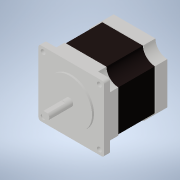
# Autodesk Inventor part: MC18_Motor
Saved by Autodesk Inventor 2021 (Build 250183000, 183)
## iProperties
Created: 2020-01-08
Part Number: MC18_Motor
Material: Generisch
Document SubType Name: Modeling
Designer: kaebi
Density: 1 g/cm^3
Appearance: Vorgabe
Description: Schrittmotor M-2222-3.0S
Stock Number: -
Author: kaebi
Autodesk Inventor part; units mm, degrees
ref_plane "YZ Plane" through (0, 0, 0) normal (1, 0, 0) x (0, 1, 0)
ref_plane "XZ Plane" through (0, 0, 0) normal (0, 1, 0) x (-1, 0, 0)
ref_plane "XY Plane" through (0, 0, 0) normal (0, 0, 1) x (1, 0, 0)
sketch "Skizze1" plane through (0, 0, 0) normal (0, 0, 1) x (1, 0, 0)
  line L0 (-27.5, -27.5) -> (27.5, -27.5)
  line L1 (27.5, -27.5) -> (27.5, 27.5)
  line L2 (27.5, 27.5) -> (-27.5, 27.5)
  line L3 (-27.5, 27.5) -> (-27.5, -27.5)
  line L4 (-27.5, -27.5) -> (27.5, 27.5) construction
  line L5 (27.5, -27.5) -> (-27.5, 27.5) construction
  point P0 (0, 0)
  dimension "d0" = 55
  dimension "d1" = 55
  constraints: 12 end point, 2 midpoint, 2 parallel, 1 horizontal, 1 perpendicular
  measures "d0" distance of L2.end L1.end
  measures "d1" distance of L1.end L0.end
extrude "Extrusion1" add sketch "Skizze1" against normal blind 12
sketch "Skizze2" plane through (0, 0, -12) normal (0, 0, -1) x (-1, 0, 0)
  line L0 (27.5, 27.5) -> (-27.5, 27.5) projected
  circle A0 centre (-27.5, 27.5) radius 10
  line L1 (27.5, -27.5) -> (27.5, 27.5) projected
  circle A1 centre (27.5, 27.5) radius 10
  circle A2 centre (27.5, -27.5) radius 10
  circle A3 centre (-27.5, -27.5) radius 10
  point P0 (0, 0)
  dimension "d4" = 20
  constraints: 4 centre point, 3 coincident, 3 equal radius
  measures "d4" diameter of A0
extrude "Extrusion2" cut sketch "Skizze2" against normal blind 7
sketch "Skizze3" plane through (0, 0, -12) normal (0, 0, -1) x (-1, 0, 0)
  arc A0 (27.5, -17.5) -> (17.5, -27.5) centre (27.5, -27.5) ccw projected
  line L0 (27.5, -17.5) -> (27.5, 17.5) projected
  arc A1 (17.5, 27.5) -> (27.5, 17.5) centre (27.5, 27.5) ccw projected
  line L1 (17.5, 27.5) -> (-17.5, 27.5) projected
  arc A2 (-27.5, 17.5) -> (-17.5, 27.5) centre (-27.5, 27.5) ccw projected
  line L2 (-27.5, 17.5) -> (-27.5, -17.5) projected
  arc A3 (-17.5, -27.5) -> (-27.5, -17.5) centre (-27.5, -27.5) ccw projected
  line L3 (-17.5, -27.5) -> (17.5, -27.5) projected
  line L4 (-17.0119, 27) -> (17.0119, 27)
  arc A4 (17.0119, 27) -> (27, 17.0119) centre (27.5, 27.5) ccw
  line L5 (27, 17.0119) -> (27, -17.0119)
  arc A5 (27, -17.0119) -> (17.0119, -27) centre (27.5, -27.5) ccw
  line L6 (17.0119, -27) -> (-17.0119, -27)
  arc A6 (-17.0119, -27) -> (-27, -17.0119) centre (-27.5, -27.5) ccw
  line L7 (-27, -17.0119) -> (-27, 17.0119)
  arc A7 (-27, 17.0119) -> (-17.0119, 27) centre (-27.5, 27.5) ccw
  point P0 (0, 0)
  dimension "d7" = 0.5
  constraints: 8 end point, 8 point on circle, 4 centre point, 7 other
  measures "d7" distance between parallel lines of L1 L4
extrude "Extrusion3" add sketch "Skizze3" along normal blind 31 contours L4 A4 L5 A5 L6 A6 L7 A7
sketch "Skizze4" plane through (0, 0, -43) normal (0, 0, -1) x (-1, 0, 0)
  arc A0 (17.0119, 27) -> (27, 17.0119) centre (27.5, 27.5) ccw projected
  line L0 (27, 17.0119) -> (27, -17.0119) projected
  arc A1 (27, -17.0119) -> (17.0119, -27) centre (27.5, -27.5) ccw projected
  line L1 (17.0119, -27) -> (-17.0119, -27) projected
  arc A2 (-17.0119, -27) -> (-27, -17.0119) centre (-27.5, -27.5) ccw projected
  line L2 (-27, -17.0119) -> (-27, 17.0119) projected
  arc A3 (-27, 17.0119) -> (-17.0119, 27) centre (-27.5, 27.5) ccw projected
  line L3 (-17.0119, 27) -> (17.0119, 27) projected
  arc A4 (27.5, -17.5) -> (17.5, -27.5) centre (27.5, -27.5) ccw projected
  line L4 (27.5, -17.5) -> (27.5, 17.5) projected
  arc A5 (17.5, 27.5) -> (27.5, 17.5) centre (27.5, 27.5) ccw projected
  line L5 (17.5, 27.5) -> (-17.5, 27.5) projected
  arc A6 (-27.5, 17.5) -> (-17.5, 27.5) centre (-27.5, 27.5) ccw projected
  line L6 (-27.5, 17.5) -> (-27.5, -17.5) projected
  arc A7 (-17.5, -27.5) -> (-27.5, -17.5) centre (-27.5, -27.5) ccw projected
  line L7 (-17.5, -27.5) -> (17.5, -27.5) projected
  point P0 (0, 0)
extrude "Extrusion4" add sketch "Skizze4" along normal blind 10 contours A0 L0 A1 L1 A2 L2 A3 L3 | A4 L7 A7 L6 A6 L5 A5 L4
sketch "Skizze6" plane through (0, 0, 0) normal (0, 0, 1) x (1, 0, 0)
  line L0 (-23.55, -23.55) -> (23.55, -23.55)
  line L1 (23.55, -23.55) -> (23.55, 23.55)
  line L2 (23.55, 23.55) -> (-23.55, 23.55)
  line L3 (-23.55, 23.55) -> (-23.55, -23.55)
  line L4 (-23.55, -23.55) -> (23.55, 23.55) construction
  line L5 (23.55, -23.55) -> (-23.55, 23.55) construction
  circle A0 centre (-23.55, 23.55) radius 2
  circle A1 centre (23.55, 23.55) radius 2
  circle A2 centre (23.55, -23.55) radius 2
  circle A3 centre (-23.55, -23.55) radius 2
  point P0 (0, 0)
  dimension "d12" = 4
  dimension "d13" = 47.1
  dimension "d14" = 47.1
  constraints: 12 end point, 4 centre point, 4 coincident, 3 equal radius, 2 midpoint, 2 parallel, 1 horizontal, 1 perpendicular
  measures "d12" diameter of A0
  measures "d13" distance of L1.end L2.end
  measures "d14" distance of L0.end L1.end
extrude "Extrusion5" cut sketch "Skizze6" along normal through all both and the other way through all contours L3 A3 L0 | L0 A3 L3 | A2 L1 L0 | L0 L1 A2 | A0 L2 L3 | L3 L2 A0 | A1 L2 L1 | L1 L2 A1
fillet "Rundung1" radius 2 4 edges at (27.5, 27.5, -2.5) (-27.5, 27.5, -2.5) (27.5, -27.5, -2.5) (-27.5, -27.5, -2.5)
sketch "Skizze7" plane through (0, 0, 0) normal (0, 0, 1) x (1, 0, 0)
  circle A0 centre (0, 0) radius 19.05
  dimension "d18" = 38.1
  constraints: 1 centre point, 1 coincident
  measures "d18" diameter of A0
extrude "Extrusion6" add sketch "Skizze7" along normal blind 1.6
sketch "Skizze8" plane through (0, 0, 1.6) normal (0, 0, 1) x (1, 0, 0)
  circle A0 centre (0, 0) radius 3.175
  dimension "d21" = 6.35
  constraints: 1 centre point, 1 coincident
  measures "d21" diameter of A0
extrude "Extrusion7" add sketch "Skizze8" along normal blind 20
sketch "Skizze9" plane through (0, 0, 21.6) normal (0, 0, 1) x (1, 0, 0)
  line L0 (-1.7861, 2.625) -> (1.7861, 2.625)
  line L1 (1.7861, 2.625) -> (1.7861, 3.175)
  line L2 (1.7861, 3.175) -> (-1.7861, 3.175)
  line L3 (-1.7861, 3.175) -> (-1.7861, 2.625)
  circle A0 centre (0, 0) radius 3.175 projected
  point P0 (0, 3.175)
  dimension "d29" = 5.8
  constraints: 8 end point, 2 parallel, 2 point on circle, 1 horizontal, 1 midpoint, 1 perpendicular, 1 vertical alignment
extrude "Extrusion8" cut sketch "Skizze9" against normal blind 15 contours A0 L0 | L3 L2 A0 | A0 L2 L1 picked at (-0.4105, 2.7255)
